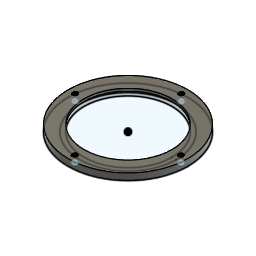
57mm speaker retainer v1.0 (Autodesk Fusion 360 design; units mm, degrees)
Autodesk Fusion 360 part; units mm, degrees
sketch "Sketch1" plane through (0, 0, 0) normal (0, 1, 0) x (1, 0, 0)
  circle A0 centre (0, 0) radius 26.5
  circle A1 centre (0, 0) radius 36
  circle A2 centre (0.0545, 32.013) radius 1.5
  circle A3 centre (-32.013, 0.0545) radius 1.5
  circle A4 centre (-0.0545, -32.013) radius 1.5
  circle A5 centre (32.013, -0.0545) radius 1.5
  circle A6 centre (0, 0) radius 29
  dimension "d1" = 53
  dimension "d2" = 72
  dimension "d3" = 3
  dimension "d5" = 360
  dimension "d8" = 58
  constraint coincident A0.centre A1.centre
  measures "d1" diameter of A0
  measures "d2" diameter of A1
  measures "d3" diameter of A2
  measures "d8" diameter of A6
extrude "Extrude1" add sketch "Sketch1" along normal blind 4 contours A1 | A6
thread "Thread1" "ISO Metric profile 3.0 M3x0.5 6H" major diameter 3.086 minor diameter 2.529 pitch 0.5 angle 60 modelled right hand crest width 0.1368 on face at (1.3344, 2.6667, -32.7952) crest through (1.319, 0.125, -32.013)
thread "Thread2" "ISO Metric profile 3.0 M3x0.5 6H" major diameter 3.086 minor diameter 2.529 pitch 0.5 angle 60 modelled right hand crest width 0.1368 on face at (32.4193, 2.6667, -1.3895) crest through (33.2775, 0.125, 0.0545)
thread "Thread3" "ISO Metric profile 3.0 M3x0.5 6H" major diameter 3.086 minor diameter 2.529 pitch 0.5 angle 60 modelled right hand crest width 0.1368 on face at (-1.4367, 2.6667, 32.5957) crest through (1.21, 0.125, 32.013)
thread "Thread4" "ISO Metric profile 3.0 M3x0.5 6H" major diameter 3.086 minor diameter 2.529 pitch 0.5 angle 60 modelled right hand crest width 0.1368 on face at (-30.5149, 2.6667, 0.0203) crest through (-30.7485, 0.125, -0.0545)
extrude "Extrude2" cut sketch "Sketch1" along normal blind 2.5 contours A6
